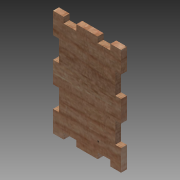
# Autodesk Inventor part: holder_ceil_plate
Saved by Autodesk Inventor 2015 (Build 190159000, 159)
## iProperties
Created: 2014-01-06
Part Number: holder_ceil_plate
Material: Wood (Birch)
Document SubType Name: Modeling
Designer: aoki
Density: 1 g/cm^3
Appearance: Birch - Natural Polished
Author: aoki
Autodesk Inventor part; units mm, degrees
ref_plane "YZ Plane" through (0, 0, 0) normal (1, 0, 0) x (0, 1, 0)
ref_plane "XZ Plane" through (0, 0, 0) normal (0, 1, 0) x (-1, 0, 0)
ref_plane "XY Plane" through (0, 0, 0) normal (0, 0, 1) x (1, 0, 0)
sketch "Block1" plane through (0, 0, 0) normal (0, 0, 1) x (1, 0, 0)
  line L0 (-10.1, 50.1) -> (-10.1, 41.1)
  line L1 (-10.1, 41.1) -> (-21.9, 41.1)
  line L2 (-21.9, 41.1) -> (-21.9, 50.1)
  line L3 (-21.9, 50.1) -> (-35.6, 50.1)
  line L4 (-35.6, 50.1) -> (-35.6, 29.9)
  line L5 (-35.6, 29.9) -> (-26.6, 29.9)
  line L6 (-26.6, 29.9) -> (-26.6, 10.1)
  line L7 (-26.6, 10.1) -> (-35.6, 10.1)
  line L8 (-35.6, 10.1) -> (-35.6, -10.1)
  line L9 (-35.6, -10.1) -> (-26.6, -10.1)
  line L10 (-26.6, -10.1) -> (-26.6, -29.9)
  line L11 (-26.6, -29.9) -> (-35.6, -29.9)
  line L12 (-35.6, -29.9) -> (-35.6, -50.1)
  line L13 (-35.6, -50.1) -> (-21.9, -50.1)
  line L14 (-21.9, -50.1) -> (-21.9, -41.1)
  line L15 (-21.9, -41.1) -> (-10.1, -41.1)
  line L16 (-10.1, -41.1) -> (-10.1, -50.1)
  line L17 (-10.1, -50.1) -> (10.1, -50.1)
  line L18 (10.1, -50.1) -> (10.1, -41.1)
  line L19 (10.1, -41.1) -> (21.9, -41.1)
  line L20 (21.9, -41.1) -> (21.9, -50.1)
  line L21 (21.9, -50.1) -> (35.6, -50.1)
  line L22 (35.6, -50.1) -> (35.6, -29.9)
  line L23 (35.6, -29.9) -> (26.6, -29.9)
  line L24 (26.6, -29.9) -> (26.6, -10.1)
  line L25 (26.6, -10.1) -> (35.6, -10.1)
  line L26 (35.6, -10.1) -> (35.6, 10.1)
  line L27 (35.6, 10.1) -> (26.6, 10.1)
  line L28 (26.6, 10.1) -> (26.6, 29.9)
  line L29 (26.6, 29.9) -> (35.6, 29.9)
  line L30 (35.6, 29.9) -> (35.6, 50.1)
  line L31 (35.6, 50.1) -> (21.9, 50.1)
  line L32 (21.9, 50.1) -> (21.9, 41.1)
  line L33 (21.9, 41.1) -> (10.1, 41.1)
  line L34 (10.1, 41.1) -> (10.1, 50.1)
  line L35 (10.1, 50.1) -> (-10.1, 50.1)
  point P0 (0, 0)
sketch "Block2" plane through (0, 0, 0) normal (0, 0, 1) x (1, 0, 0)
  line L0 (-10.2, 50.2) -> (-10.2, 41.2)
  line L1 (-10.2, 41.2) -> (-21.8, 41.2)
  line L2 (-21.8, 41.2) -> (-21.8, 50.2)
  line L3 (-21.8, 50.2) -> (-35.7, 50.2)
  line L4 (-35.7, 50.2) -> (-35.7, 29.8)
  line L5 (-35.7, 29.8) -> (-26.7, 29.8)
  line L6 (-26.7, 29.8) -> (-26.7, 10.2)
  line L7 (-26.7, 10.2) -> (-35.7, 10.2)
  line L8 (-35.7, 10.2) -> (-35.7, -10.2)
  line L9 (-35.7, -10.2) -> (-26.7, -10.2)
  line L10 (-26.7, -10.2) -> (-26.7, -29.8)
  line L11 (-26.7, -29.8) -> (-35.7, -29.8)
  line L12 (-35.7, -29.8) -> (-35.7, -50.2)
  line L13 (-35.7, -50.2) -> (-21.8, -50.2)
  line L14 (-21.8, -50.2) -> (-21.8, -41.2)
  line L15 (-21.8, -41.2) -> (-10.2, -41.2)
  line L16 (-10.2, -41.2) -> (-10.2, -50.2)
  line L17 (-10.2, -50.2) -> (10.2, -50.2)
  line L18 (10.2, -50.2) -> (10.2, -41.2)
  line L19 (10.2, -41.2) -> (21.8, -41.2)
  line L20 (21.8, -41.2) -> (21.8, -50.2)
  line L21 (21.8, -50.2) -> (35.7, -50.2)
  line L22 (35.7, -50.2) -> (35.7, -29.8)
  line L23 (35.7, -29.8) -> (26.7, -29.8)
  line L24 (26.7, -29.8) -> (26.7, -10.2)
  line L25 (26.7, -10.2) -> (35.7, -10.2)
  line L26 (35.7, -10.2) -> (35.7, 10.2)
  line L27 (35.7, 10.2) -> (26.7, 10.2)
  line L28 (26.7, 10.2) -> (26.7, 29.8)
  line L29 (26.7, 29.8) -> (35.7, 29.8)
  line L30 (35.7, 29.8) -> (35.7, 50.2)
  line L31 (35.7, 50.2) -> (21.8, 50.2)
  line L32 (21.8, 50.2) -> (21.8, 41.2)
  line L33 (21.8, 41.2) -> (10.2, 41.2)
  line L34 (10.2, 41.2) -> (10.2, 50.2)
  line L35 (10.2, 50.2) -> (-10.2, 50.2)
  point P0 (0, 0)
sketch "Block3" plane through (0, 0, 0) normal (0, 0, 1) x (1, 0, 0)
  line L0 (-10.1, 50.1) -> (-10.1, 41.1)
  line L1 (-10.1, 41.1) -> (-21.9, 41.1)
  line L2 (-21.9, 41.1) -> (-21.9, 50.1)
  line L3 (-21.9, 50.1) -> (-35.6, 50.1)
  line L4 (-35.6, 50.1) -> (-35.6, 29.9)
  line L5 (-35.6, 29.9) -> (-26.6, 29.9)
  line L6 (-26.6, 29.9) -> (-26.6, 10.1)
  line L7 (-26.6, 10.1) -> (-35.6, 10.1)
  line L8 (-35.6, 10.1) -> (-35.6, -10.1)
  line L9 (-35.6, -10.1) -> (-26.6, -10.1)
  line L10 (-26.6, -10.1) -> (-26.6, -29.9)
  line L11 (-26.6, -29.9) -> (-35.6, -29.9)
  line L12 (-35.6, -29.9) -> (-35.6, -50.1)
  line L13 (-35.6, -50.1) -> (-21.9, -50.1)
  line L14 (-21.9, -50.1) -> (-21.9, -41.1)
  line L15 (-21.9, -41.1) -> (-10.1, -41.1)
  line L16 (-10.1, -41.1) -> (-10.1, -50.1)
  line L17 (-10.1, -50.1) -> (10.1, -50.1)
  line L18 (10.1, -50.1) -> (10.1, -41.1)
  line L19 (10.1, -41.1) -> (21.9, -41.1)
  line L20 (21.9, -41.1) -> (21.9, -50.1)
  line L21 (21.9, -50.1) -> (35.6, -50.1)
  line L22 (35.6, -50.1) -> (35.6, -29.9)
  line L23 (35.6, -29.9) -> (26.6, -29.9)
  line L24 (26.6, -29.9) -> (26.6, -10.1)
  line L25 (26.6, -10.1) -> (35.6, -10.1)
  line L26 (35.6, -10.1) -> (35.6, 10.1)
  line L27 (35.6, 10.1) -> (26.6, 10.1)
  line L28 (26.6, 10.1) -> (26.6, 29.9)
  line L29 (26.6, 29.9) -> (35.6, 29.9)
  line L30 (35.6, 29.9) -> (35.6, 50.1)
  line L31 (35.6, 50.1) -> (21.9, 50.1)
  line L32 (21.9, 50.1) -> (21.9, 41.1)
  line L33 (21.9, 41.1) -> (10.1, 41.1)
  line L34 (10.1, 41.1) -> (10.1, 50.1)
  line L35 (10.1, 50.1) -> (-10.1, 50.1)
  point P0 (0, 0)
sketch "Block4" plane through (0, 0, 0) normal (0, 0, 1) x (1, 0, 0)
  line L0 (-10.08, 50.08) -> (-10.08, 44.58)
  line L1 (-10.08, 44.58) -> (-21.92, 44.58)
  line L2 (-21.92, 44.58) -> (-21.92, 50.08)
  line L3 (-21.92, 50.08) -> (-32.08, 50.08)
  line L4 (-32.08, 50.08) -> (-32.08, 29.92)
  line L5 (-32.08, 29.92) -> (-26.58, 29.92)
  line L6 (-26.58, 29.92) -> (-26.58, 10.08)
  line L7 (-26.58, 10.08) -> (-32.08, 10.08)
  line L8 (-32.08, 10.08) -> (-32.08, -10.08)
  line L9 (-32.08, -10.08) -> (-26.58, -10.08)
  line L10 (-26.58, -10.08) -> (-26.58, -29.92)
  line L11 (-26.58, -29.92) -> (-32.08, -29.92)
  line L12 (-32.08, -29.92) -> (-32.08, -50.08)
  line L13 (-32.08, -50.08) -> (-21.92, -50.08)
  line L14 (-21.92, -50.08) -> (-21.92, -44.58)
  line L15 (-21.92, -44.58) -> (-10.08, -44.58)
  line L16 (-10.08, -44.58) -> (-10.08, -50.08)
  line L17 (-10.08, -50.08) -> (10.08, -50.08)
  line L18 (10.08, -50.08) -> (10.08, -44.58)
  line L19 (10.08, -44.58) -> (21.92, -44.58)
  line L20 (21.92, -44.58) -> (21.92, -50.08)
  line L21 (21.92, -50.08) -> (32.08, -50.08)
  line L22 (32.08, -50.08) -> (32.08, -29.92)
  line L23 (32.08, -29.92) -> (26.58, -29.92)
  line L24 (26.58, -29.92) -> (26.58, -10.08)
  line L25 (26.58, -10.08) -> (32.08, -10.08)
  line L26 (32.08, -10.08) -> (32.08, 10.08)
  line L27 (32.08, 10.08) -> (26.58, 10.08)
  line L28 (26.58, 10.08) -> (26.58, 29.92)
  line L29 (26.58, 29.92) -> (32.08, 29.92)
  line L30 (32.08, 29.92) -> (32.08, 50.08)
  line L31 (32.08, 50.08) -> (21.92, 50.08)
  line L32 (21.92, 50.08) -> (21.92, 44.58)
  line L33 (21.92, 44.58) -> (10.08, 44.58)
  line L34 (10.08, 44.58) -> (10.08, 50.08)
  line L35 (10.08, 50.08) -> (-10.08, 50.08)
  point P0 (0, 0)
sketch "Sketch1" plane through (0, 0, 0) normal (0, 1, 0) x (-1, 0, 0)
  line L0 (32, -50) -> (-32, -50)
  line L1 (-32, -50) -> (-32, 50)
  line L2 (-32, 50) -> (32, 50)
  line L3 (32, 50) -> (32, -50)
  line L4 (32, -50) -> (-32, 50) construction
  line L5 (-32, -50) -> (32, 50) construction
  point P0 (0, 0)
  dimension "d0" = 64
  dimension "d1" = 100
  constraints: 12 end point, 2 midpoint, 2 parallel, 1 horizontal, 1 perpendicular
  measures "d0" distance of L1.end L2.end
  measures "d1" distance of L0.end L1.end
extrude "Extrusion1" add sketch "Sketch1" along normal blind 5.5
sketch "Sketch5" plane through (0, 5.5, 0) normal (0, 1, 0) x (1, 0, 0)
  line L0 (32, 50) -> (-32, 50) projected
  line L1 (-32, 50) -> (-32, -50) projected
  line L2 (-32, 30) -> (-26.5, 30)
  line L3 (-26.5, 30) -> (-26.5, 10)
  line L4 (-26.5, 10) -> (-32, 10)
  line L5 (-32, 10) -> (-32, 30)
  line L6 (-66.1027, 0) -> (147.4162, 0) projected
  line L7 (0, 70.495) -> (0, -72.2701) projected
  line L8 (-32, -30) -> (-26.5, -30)
  line L9 (-26.5, -30) -> (-26.5, -10)
  line L10 (-26.5, -10) -> (-32, -10)
  line L11 (-32, -10) -> (-32, -30)
  line L12 (32, 30) -> (26.5, 30)
  line L13 (26.5, 30) -> (26.5, 10)
  line L14 (26.5, 10) -> (32, 10)
  line L15 (32, 10) -> (32, 30)
  line L16 (32, -30) -> (26.5, -30)
  line L17 (26.5, -30) -> (26.5, -10)
  line L18 (26.5, -10) -> (32, -10)
  line L19 (32, -10) -> (32, -30)
  point P0 (0, 0)
  dimension "d12" = 20
  dimension "d13" = 20
  dimension "d14" = 5.5
  constraints: 32 end point, 12 symmetric about line, 2 parallel, 1 collinear, 1 horizontal, 1 perpendicular
  measures "d12" distance between parallel lines of L0 L2
  measures "d13" distance of L2.end L3.end
  measures "d14" distance of L3.end L4.end
extrude "Extrusion3" cut sketch "Sketch5" against normal through all contours L10 L9 L8 L1 | L2 L3 L4 L1 | L15 L14 L13 L12 | L16 L17 L18 L19
sketch "Sketch6" plane through (0, 5.5, 0) normal (0, 1, 0) x (1, 0, 0)
  line L0 (32, 50) -> (-32, 50) projected
  line L1 (-66.1027, 0) -> (147.4162, 0) projected
  line L2 (0, 70.495) -> (0, -72.2701) projected
  line L3 (-22, 50) -> (-10, 50)
  line L4 (-10, 50) -> (-10, 44.5)
  line L5 (-10, 44.5) -> (-22, 44.5)
  line L6 (-22, 44.5) -> (-22, 50)
  line L7 (22, 50) -> (10, 50)
  line L8 (10, 50) -> (10, 44.5)
  line L9 (10, 44.5) -> (22, 44.5)
  line L10 (22, 44.5) -> (22, 50)
  line L11 (-22, -50) -> (-10, -50)
  line L12 (-10, -50) -> (-10, -44.5)
  line L13 (-10, -44.5) -> (-22, -44.5)
  line L14 (-22, -44.5) -> (-22, -50)
  line L15 (10, -44.5) -> (22, -44.5)
  line L16 (22, -50) -> (10, -50)
  line L17 (10, -50) -> (10, -44.5)
  line L18 (22, -44.5) -> (22, -50)
  point P0 (0, 0)
  dimension "d17" = 5.5
  dimension "d18" = 12
  dimension "d19" = 20
  constraints: 32 end point, 12 symmetric about line, 2 parallel, 1 horizontal, 1 perpendicular, 1 point on line
  measures "d17" distance of L3.end L4.end
  measures "d18" distance of L4.end L5.end
  measures "d19" distance between parallel lines of L8 L4
extrude "Extrusion4" cut sketch "Sketch6" against normal through all
equation "\"d2\" = Wt"
equation "\"d14\" = Wt"
equation "\"d15\" = Wt"
equation "\"d17\" = Wt"
equation "\"d20\" = Wt"
equation "\"Wt\" = 5.5"
body "Solid1"
